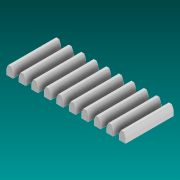
# Autodesk Inventor part: rack_enkelvoudig
Saved by Autodesk Inventor 2020.3 (Build 243373000, 373)
## iProperties
Created: 2020-05-26
Part Number: rack_enkelvoudig
Material: Generic
Document SubType Name: Modeling
Designer: Svend
Density: 1 g/cm^3
Appearance: Default
Author: Svend
Autodesk Inventor part; units mm, degrees
ref_plane "YZ Plane" through (0, 0, 0) normal (1, 0, 0) x (0, 1, 0)
ref_plane "XZ Plane" through (0, 0, 0) normal (0, 1, 0) x (-1, 0, 0)
ref_plane "XY Plane" through (0, 0, 0) normal (0, 0, 1) x (1, 0, 0)
sketch "Sketch1" plane through (0, 0, 0) normal (0, 0, 1) x (1, 0, 0)
  spline S0 degree 3 poles (1.427833, 2.329374) (1.438406, 2.311121) (1.464006, 2.266243) (1.503081, 2.195018) (1.544186, 2.116405) (1.582371, 2.039677) (1.617729, 1.96492) (1.650354, 1.892214) (1.680343, 1.821639) (1.707795, 1.753269) (1.73281, 1.687176) (1.755491, 1.623429) (1.775942, 1.562095) (1.794269, 1.503235) (1.810579, 1.446909) (1.824982, 1.393174) (1.837588, 1.34208) (1.848509, 1.293679) (1.857857, 1.248015) (1.865747, 1.205131) (1.872295, 1.165065) (1.877615, 1.127854) (1.881825, 1.093529) (1.885042, 1.062118) (1.887387, 1.033646) (1.888974, 1.008135) (1.904089, 0.652654) (1.739325, 0.300573) (2.151053, 0) knots 0.46137242 0.46137242 0.46137242 0.46137242 0.47526399 0.4953967 0.51486932 0.53368185 0.5518343 0.56932665 0.58615892 0.60233109 0.61784318 0.63269518 0.64688709 0.66041891 0.67329065 0.68550229 0.69705385 0.70794531 0.71817669 0.72774798 0.73665918 0.74491029 0.75250131 0.75943225 0.76570309 0.77131385 0.77626451 1 1 1 1
  arc A0 (1.427833, 2.329374) -> (0.723221, 2.329374) centre (1.075527, -6.562449) ccw
  spline S1 degree 3 poles (0, 0) (0.411732, 0.300572) (0.250534, 0.645031) (0.261165, 0.984596) (0.261401, 0.99211) (0.26172, 0.999621) (0.262108, 1.007129) (0.262549, 1.015638) (0.263078, 1.024141) (0.263687, 1.032639) (0.264368, 1.042137) (0.26515, 1.051628) (0.266021, 1.06111) (0.266984, 1.071591) (0.268056, 1.082061) (0.269228, 1.09252) (0.270512, 1.103975) (0.271915, 1.115417) (0.273428, 1.126844) (0.275072, 1.139265) (0.276846, 1.151669) (0.278738, 1.164054) (0.280781, 1.177431) (0.282964, 1.190786) (0.285275, 1.204118) (0.287756, 1.218439) (0.290386, 1.232734) (0.293154, 1.247002) (0.296113, 1.262253) (0.299229, 1.277475) (0.302492, 1.292664) (0.305966, 1.308834) (0.309606, 1.324968) (0.313402, 1.341065) (0.317429, 1.358138) (0.321631, 1.375169) (0.325998, 1.392157) (0.330614, 1.410117) (0.335415, 1.428029) (0.34039, 1.445892) (0.345634, 1.464721) (0.351071, 1.483496) (0.35669, 1.502217) (0.362597, 1.521897) (0.368706, 1.541517) (0.375006, 1.561076) (0.381613, 1.581588) (0.38843, 1.602033) (0.395446, 1.622409) (0.402788, 1.643733) (0.410348, 1.664982) (0.418116, 1.686155) (0.426228, 1.708269) (0.434567, 1.7303) (0.44312, 1.752247) (0.452037, 1.775128) (0.461187, 1.797918) (0.47056, 1.820616) (0.480316, 1.844241) (0.490312, 1.867766) (0.500538, 1.891191) (0.511165, 1.915535) (0.52204, 1.93977) (0.533152, 1.963896) (0.544683, 1.988932) (0.556469, 2.013852) (0.568498, 2.038652) (0.580965, 2.064355) (0.593693, 2.089931) (0.606671, 2.115379) (0.620105, 2.141721) (0.633807, 2.167925) (0.647765, 2.193992) (0.662196, 2.220943) (0.676901, 2.247748) (0.691868, 2.274405) (0.702195, 2.292798) (0.712647, 2.311121) (0.723221, 2.329374) knots 0 0 0 0 0.22373549 0.22373549 0.22373549 0.22868615 0.22868615 0.22868615 0.23429691 0.23429691 0.23429691 0.24056775 0.24056775 0.24056775 0.24749869 0.24749869 0.24749869 0.25508971 0.25508971 0.25508971 0.26334082 0.26334082 0.26334082 0.27225202 0.27225202 0.27225202 0.28182331 0.28182331 0.28182331 0.29205469 0.29205469 0.29205469 0.30294615 0.30294615 0.30294615 0.31449771 0.31449771 0.31449771 0.32670935 0.32670935 0.32670935 0.33958109 0.33958109 0.33958109 0.35311291 0.35311291 0.35311291 0.36730482 0.36730482 0.36730482 0.38215682 0.38215682 0.38215682 0.39766891 0.39766891 0.39766891 0.41384108 0.41384108 0.41384108 0.43067335 0.43067335 0.43067335 0.4481657 0.4481657 0.4481657 0.46631815 0.46631815 0.46631815 0.48513068 0.48513068 0.48513068 0.5046033 0.5046033 0.5046033 0.52473601 0.52473601 0.52473601 0.53862758 0.53862758 0.53862758 0.53862758
  line L0 (4.211664, 0) -> (-4.211664, 0)
  line L1 (0.260648, 0.95) -> (1.890408, 0.95)
  line L2 (1.890408, 0.95) -> (1.890408, 0)
  line L3 (0.260648, 0.95) -> (0.260648, 0)
  line L4 (0.416403, 1.681475) -> (1.734652, 1.681475)
  line L5 (0, 0) -> (20, 0)
  dimension "d2" = 0.95
  dimension "d3" = 8.8988
  dimension "d4" = 2.32937
  dimension "d5" = 2.32937
  dimension "d6" = 0.72322
  dimension "d7" = 0.70461
  dimension "d8" = 0.26065
  dimension "d9" = 1.62976
  dimension "d10" = 20
  constraints: 12 end point, 5 coincident, 4 horizontal, 2 perpendicular, 2 point on circle, 2 point on line, 1 centre point, 1 midpoint, 8 other
  measures "d2" distance between parallel lines of L0 L1
  measures "d3" radius of A0
  measures "d4" distance from line of L0 A0.start
  measures "d5" distance from line of L0 A0.end
  measures "d6" horizontal distance of point (0, 0) point (0.723, 2.329)
  measures "d7" distance of A0.end point (1.428, 2.329)
  measures "d8" horizontal distance of point (0, 0) point (0.261, 0.95)
  measures "d9" distance of point (0.261, 0.95) point (1.89, 0.95)
  measures "d10" distance of L5.start L5.end
extrude "Extrusion1" add sketch "Sketch1" along normal blind 12 contours S0 L4 S1 A0 | S0 L1 S1 L4 | L2 S0 | S0 L2 L0 L3 S1 L1 | S1 L3
pattern_linear "Rectangular Pattern1" count 10 spacing 3.136 along (1, 0, 0) of "Extrusion1"
equation "\"d5\" = d4"
body "Solid1"
